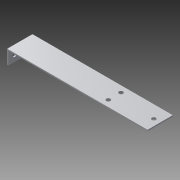
# Autodesk Inventor part: 爪＿2
Saved by Autodesk Inventor 2015 (Build 190159000, 159)
## iProperties
Created: 2015-05-18
Part Number: 爪＿2
Material: アルミニウム 6061
Document SubType Name: Modeling
Designer: kenta
Density: 2.7 g/cm^3
Appearance: アルミニウム - フラット
Mass: 6.42543 g
Surface Area: 50.9184 cm^2
Volume: 2.37979 cm^3
Author: kenta
Autodesk Inventor part; units mm, degrees
ref_plane "YZ Plane" through (0, 0, 0) normal (1, 0, 0) x (0, 1, 0)
ref_plane "XZ Plane" through (0, 0, 0) normal (0, 1, 0) x (-1, 0, 0)
ref_plane "XY Plane" through (0, 0, 0) normal (0, 0, 1) x (1, 0, 0)
sketch "スケッチ1" plane through (0, 0, 0) normal (0, 0, 1) x (1, 0, 0)
  line L0 (-60, 10) -> (60, 10)
  line L1 (60, 10) -> (60, -10)
  line L2 (60, -10) -> (-60, -10)
  line L3 (-60, -10) -> (-60, 10)
  line L4 (-60, 10) -> (60, -10) construction
  line L5 (60, 10) -> (-60, -10) construction
  point P0 (0, 0)
  dimension "d0" = 120
  dimension "d1" = 20
  constraints: 12 end point, 2 midpoint, 2 parallel, 1 horizontal, 1 perpendicular
  measures "d0" distance of L1.end L2.end
  measures "d1" distance of L0.end L1.end
extrude "押し出し1" add sketch "スケッチ1" along normal blind 1
sketch "スケッチ2" plane through (0, 0, 1) normal (0, 0, 1) x (1, 0, 0)
  line L0 (60, -10) -> (60, 10) projected
  line L1 (60, 10) -> (-60, 10) projected
  line L2 (-60, 10) -> (-60, -10) projected
  line L3 (-60, -10) -> (60, -10) projected
  point P0 (0, 0)
  point P1 (14, 5)
  point P2 (14, -5)
  point P3 (45, 0)
  dimension "d4" = 15
  dimension "d5" = 10
  dimension "d7" = 46
  dimension "d8" = 5
  dimension "d9" = 5
  constraints: 1 vertical alignment
  measures "d4" distance from line of L0 point (45, 0)
  measures "d5" distance from line of point (45, 0) L1
  measures "d7" distance from line of point (14, 5) L0
  measures "d8" distance from line of point (14, 5) L1
  measures "d9" distance from line of point (14, -5) L3
hole "穴1" at (14, 5, 1) at (14, -5, 1) at (45, 0, 1) direction (0, 0, -1) diameter 3.2 end through all
sketch "スケッチ3" plane through (0, 0, 1) normal (0, 0, 1) x (1, 0, 0)
  line L0 (-60, 10) -> (-61, 10)
  line L1 (-61, 10) -> (-61, -10)
  line L2 (-61, -10) -> (-60, -10)
  line L3 (-60, -10) -> (-60, 10)
  point P0 (0, 0)
  dimension "d17" = 1
  dimension "d18" = 20
  constraints: 8 end point, 2 parallel, 1 horizontal, 1 perpendicular
  measures "d17" distance of L2.end L1.end
  measures "d18" distance of L1.end L0.end
extrude "押し出し2" add sketch "スケッチ3" against normal blind 11
sketch "スケッチ4" plane through (-60, -10, 0) normal (1, 0, 0) x (0, 0, -1)
  line L0 (10, 20) -> (10, 0) projected
  line L1 (0, 20) -> (10, 20) projected
  line L2 (0, 0) -> (10, 0) projected
  point P0 (0, 10)
  point P1 (5, 15)
  point P2 (5, 5)
  dimension "d21" = 5
  dimension "d22" = 5
  dimension "d30" = 5
  dimension "d31" = 5
  dimension "d32" = 10
  measures "d21" distance from line of point (5, 15) L0
  measures "d22" distance from line of point (5, 15) L1
  measures "d30" distance from line of point (5, 5) L2
  measures "d31" distance from line of point (5, 5) L0
  measures "d32" distance of point (5, 15) point (5, 5)
hole "穴2" at (-60, 5, -5) at (-60, -5, -5) direction (-1, 0, 0) diameter 3.2 end through all
sketch "スケッチ5" plane through (0, 0, 1) normal (0, 0, 1) x (1, 0, 0)
  line L0 (-61, -10) -> (60, -10) projected
  line L1 (60, 10) -> (50, 10)
  line L2 (50, 10) -> (50, -10)
  line L3 (50, -10) -> (60, -10)
  line L4 (60, -10) -> (60, 10)
  point P0 (0, 0)
  dimension "d33" = 10
  constraints: 8 end point, 2 parallel, 1 horizontal, 1 perpendicular, 1 point on line
  measures "d33" distance of L1.start L1.end
extrude "押し出し3" cut sketch "スケッチ5" against normal blind 10
